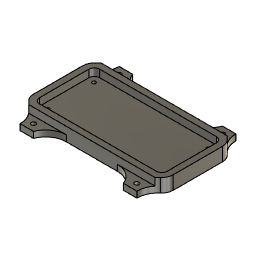
amod3-electronics_platform v9 (Autodesk Fusion 360 archive; units mm, degrees)
design "amod3-px_holder"
Autodesk Fusion 360 part; units mm, degrees
sketch "Sketch1" plane through (0, 0, 0) normal (0, 0, 1) x (1, 0, 0)
  line L0 (-21, 0) -> (65.86, 0)
  line L1 (69.86, 4) -> (69.86, 40.69)
  line L2 (65.86, 44.69) -> (-21, 44.69)
  line L3 (-25, 40.69) -> (-25, 4)
  arc A0 (-21, 44.69) -> (-25, 40.69) centre (-21, 40.69) ccw
  arc A1 (-25, 4) -> (-21, 0) centre (-21, 4) ccw
  arc A2 (69.86, 40.69) -> (65.86, 44.69) centre (65.86, 40.69) ccw
  arc A3 (65.86, 0) -> (69.86, 4) centre (65.86, 4) ccw
  line L4 (-25, 44.69) -> (69.86, 0)
  line L5 (69.86, 0) -> (69.86, 44.69)
  line L6 (69.86, 44.69) -> (-25, 0)
  line L7 (64.93, 5.145) -> (-20.07, 5.145)
  line L8 (-20.07, 5.145) -> (-20.07, 39.545)
  line L9 (-20.07, 39.545) -> (64.93, 39.545)
  line L10 (64.93, 39.545) -> (64.93, 5.145)
  line L11 (64.93, 5.145) -> (-20.07, 39.545) construction
  line L12 (-20.07, 5.145) -> (64.93, 39.545) construction
  circle A4 centre (-20.07, 39.545) radius 1.35
  circle A5 centre (64.93, 39.545) radius 1.35
  circle A6 centre (-20.07, 5.145) radius 1.35
  circle A7 centre (64.93, 5.145) radius 1.35
  line L13 (-29.5, 40.69) -> (-29.5, 4)
  arc A8 (-29.5, 4) -> (-21, -4.5) centre (-21, 4) ccw
  line L14 (-21, -4.5) -> (65.86, -4.5)
  arc A9 (65.86, -4.5) -> (74.36, 4) centre (65.86, 4) ccw
  line L15 (74.36, 4) -> (74.36, 40.69)
  arc A10 (74.36, 40.69) -> (65.86, 49.19) centre (65.86, 40.69) ccw
  line L16 (65.86, 49.19) -> (-21, 49.19)
  arc A11 (-21, 49.19) -> (-29.5, 40.69) centre (-21, 40.69) ccw
  circle A12 centre (-20.07, 5.145) radius 2.6
  circle A13 centre (64.93, 5.145) radius 2.6
  circle A14 centre (-20.07, 39.545) radius 2.6
  circle A15 centre (64.93, 39.545) radius 2.6
  line L17 (-21, -4.5) -> (-11, -4.5)
  line L18 (-11, -4.5) -> (-11, -14.5)
  line L19 (-11, -14.5) -> (-21, -14.5)
  line L20 (-21, -14.5) -> (-21, -4.5)
  line L21 (-11, -4.5) -> (-21, -4.5)
  line L22 (65.86, -4.5) -> (55.86, -4.5)
  line L23 (65.86, -4.5) -> (65.86, -14.5)
  line L24 (65.86, -14.5) -> (55.86, -14.5)
  line L25 (55.86, -14.5) -> (55.86, -4.5)
  line L26 (-11, 59.19) -> (-21, 59.19)
  line L27 (-11, 59.19) -> (-11, 49.19)
  line L28 (-11, 49.19) -> (-21, 49.19)
  line L29 (-21, 49.19) -> (-21, 59.19)
  line L30 (65.86, 59.19) -> (55.86, 59.19)
  line L31 (65.86, 59.19) -> (65.86, 49.19)
  line L32 (65.86, 49.19) -> (55.86, 49.19)
  line L33 (55.86, 49.19) -> (55.86, 59.19)
  point P0 (-25, 0)
  point P1 (69.86, 0)
  point P2 (-25, 44.69)
  point P3 (22.43, 22.345)
  dimension "d1" = 94.86
  dimension "d2" = 44.69
  dimension "d3" = 4
  dimension "d4" = 4
  dimension "d5" = 4
  dimension "d6" = 4
  dimension "d7" = 85
  dimension "d8" = 34.4
  dimension "d9" = 2.7
  dimension "d12" = 85
  dimension "d13" = -34.4
  dimension "d14" = 4.5
  dimension "d19" = 5.2
  dimension "d22" = 85
  dimension "d23" = 34.4
  dimension "d28" = 10
  dimension "d29" = 10
  dimension "d32" = 76.86
  dimension "d33" = 63.69
  constraint horizontal L0
  constraint vertical L1
  constraint horizontal L2
  constraint vertical L3
  constraint coincident P2 L2
  constraint coincident P2 L3
  constraint tangent L2 A0
  constraint tangent L3 A0
  constraint coincident P0 L0
  constraint coincident P0 L3
  constraint tangent L0 A1
  constraint tangent L3 A1
  constraint tangent L1 A2
  constraint tangent L2 A2
  constraint coincident P1 L0
  constraint coincident P1 L1
  constraint tangent L0 A3
  constraint tangent L1 A3
  constraint coincident P2 L4.start
  constraint coincident P1 L4.end
  constraint vertical L5
  constraint coincident P0 L6.end
  constraint horizontal L7
  constraint perpendicular L7 L8
  constraint parallel L7 L9
  constraint parallel L8 L10
  constraint coincident L11 P3
  constraint coincident L12 P3
  constraint midpoint L4 P3
  constraint coincident L8.end L9.start
  constraint concentric A6 A12
  constraint horizontal L17
  constraint vertical L18
  constraint horizontal L19
  constraint vertical L20
  measures "d1" distance of P0 L4.end
  measures "d2" distance of P0 P2
  measures "d3" radius of A0
  measures "d4" radius of A1
  measures "d5" radius of A2
  measures "d6" radius of A3
  measures "d7" distance of L8.end L9.end
  measures "d8" distance of L7.end L8.end
  measures "d9" diameter of A4
  measures "d19" diameter of A12
  measures "d28" distance of A8.end L17.end
  measures "d29" distance of A8.end L19.end
extrude "Extrude1" add sketch "Sketch1" along normal blind 10 contours A3 L4 L5 | A2 L5 L6 | L13 A8 L14 A9 L15 A10 L16 A11 L17 L21 L22 L28 L32
extrude "Extrude2" add sketch "Sketch1" along normal blind 3 contours L0 A1 A3 L4 L6 L7 A12 A13 | L3 A0 A1 L4 L6 L8 A12 A14 | L1 A2 A3 L4 L5 L6 L10 A13 A15 | L6 L7 L8 A6 A12 | L6 A12 | L4 A13 | L4 L7 L10 A7 A13 | L6 L7 A12 | L7 L8 A6 A12 | L4 L6 L7 L8 L9 A12 A14 | L4 L7 A13 | L2 A0 A2 L4 L6 L9 A14 A15 | L4 L6 L7 | L4 L8 L9 A4 A14 | L8 L9 A4 A14 | L4 L6 L7 L9 L10 A13 A15 | L7 L10 A7 A13 | L4 A14 | L4 L6 L9 | L4 L9 A14 | L6 L9 L10 A5 A15 | L6 A15 | L9 L10 A5 A15 | L6 L9 A15
sketch "Sketch2" plane through (0, 0, 0) normal (0, 0, 1) x (1, 0, 0)
extrude "Extrude3" cut sketch "Sketch1" along normal blind 2.5 contours L6 L7 L8 A6 A12 | L4 L7 L10 A7 A13 | L7 L8 A6 A12 | L4 L8 L9 A4 A14 | L8 L9 A4 A14 | L7 L10 A7 A13 | L6 L9 L10 A5 A15 | L9 L10 A5 A15
extrude "Extrude4" add 1 faces at (36.1652, 16.8113, 3) along direction (0, 0, 1) blind 1.5
extrude "Extrude5" add sketch "Sketch1" along normal blind 4.5 contours L16 L26 L27 L28 L29 | L14 L17 L18 L19 L20 L21 | L16 L30 L31 L32 L33 | L14 L22 L23 L24 L25
sketch "Sketch3" plane through (0, 0, 0) normal (0, 0, -1) x (1, 0, 0)
  line L0 (-18.5378, -41.6456) -> (-19.4259, -42.064)
  arc A0 (-18.5378, -41.6456) -> (-19.4259, -42.064) centre (-20.07, -39.545) ccw
  line L1 (64.2859, -42.064) -> (63.3978, -41.6456)
  arc A1 (64.2859, -42.064) -> (63.3978, -41.6456) centre (64.93, -39.545) ccw
  line L2 (-19.4259, -2.626) -> (-18.5378, -3.0444)
  arc A2 (-19.4259, -2.626) -> (-18.5378, -3.0444) centre (-20.07, -5.145) ccw
  line L3 (63.3978, -3.0444) -> (64.2859, -2.626)
  arc A3 (63.3978, -3.0444) -> (64.2859, -2.626) centre (64.93, -5.145) ccw
  arc A4 (-29.5, -40.69) -> (-21, -49.19) centre (-21, -40.69) ccw
  line L4 (-21, -49.19) -> (-21, -59.19)
  line L5 (-21, -59.19) -> (-11, -59.19)
  line L6 (-11, -59.19) -> (-11, -49.19)
  line L7 (-11, -49.19) -> (55.86, -49.19)
  line L8 (55.86, -49.19) -> (55.86, -59.19)
  line L9 (55.86, -59.19) -> (65.86, -59.19)
  line L10 (65.86, -59.19) -> (65.86, -49.19)
  arc A5 (65.86, -49.19) -> (74.36, -40.69) centre (65.86, -40.69) ccw
  line L11 (74.36, -40.69) -> (74.36, -4)
  arc A6 (74.36, -4) -> (65.86, 4.5) centre (65.86, -4) ccw
  line L12 (65.86, 4.5) -> (65.86, 14.5)
  line L13 (65.86, 14.5) -> (55.86, 14.5)
  line L14 (55.86, 14.5) -> (55.86, 4.5)
  line L15 (55.86, 4.5) -> (-11, 4.5)
  line L16 (-11, 4.5) -> (-11, 14.5)
  line L17 (-11, 14.5) -> (-21, 14.5)
  line L18 (-21, 14.5) -> (-21, 4.5)
  arc A7 (-21, 4.5) -> (-29.5, -4) centre (-21, -4) ccw
  line L19 (-29.5, -4) -> (-29.5, -40.69)
  line L20 (-21, 14.5) -> (65.86, 14.5)
  line L21 (65.86, 14.5) -> (65.86, -59.19)
  line L22 (65.86, -59.19) -> (-21, -59.19)
  line L23 (-21, -59.19) -> (-21, 14.5)
  line L24 (-11, 4.5) -> (55.86, 4.5)
  line L25 (55.86, 4.5) -> (55.86, -49.19)
  line L26 (55.86, -49.19) -> (-11, -49.19)
  line L27 (-11, -49.19) -> (-11, 4.5)
  line L28 (-11, 4.5) -> (-21, 14.5)
  line L29 (55.86, 4.5) -> (65.86, 14.5)
  line L30 (55.86, -49.19) -> (65.86, -59.19)
  line L31 (-11, -49.19) -> (-21, -59.19)
  circle A8 centre (-16, 9.5) radius 1.65
  circle A9 centre (60.86, 9.5) radius 1.65
  circle A10 centre (-16, -54.19) radius 1.65
  circle A11 centre (60.86, -54.19) radius 1.65
  dimension "d36" = 3.3
  dimension "d37" = 3.3
  dimension "d38" = 3.3
  dimension "d39" = 3.3
  constraint horizontal L20
  constraint vertical L21
  constraint horizontal L22
  constraint vertical L23
  constraint coincident L9.end L10.start
  constraint coincident L17.end L18.start
  constraint horizontal L24
  constraint vertical L25
  constraint horizontal L26
  constraint vertical L27
  constraint coincident L7.end L8.start
  constraint coincident L15.end L16.start
  constraint coincident L14.end L15.start
  constraint coincident L12.end L13.start
  constraint coincident L6.end L7.start
  constraint coincident L4.end L5.start
  constraint midpoint L28 A8.centre
  constraint midpoint L29 A9.centre
  constraint midpoint L31 A10.centre
  constraint midpoint L30 A11.centre
  measures "d36" diameter of A8
  measures "d37" diameter of A9
  measures "d38" diameter of A10
  measures "d39" diameter of A11
extrude "Extrude6" cut sketch "Sketch3" against normal blind 8.5 contours L31 A10 | L31 A10 | L28 A8 | L28 A8 | L30 A11 | L30 A11 | L29 A9 | L29 A9
fillet "Fillet1" radius 15.5 8 edges at (-21, -4.5, 2.25) (55.86, -4.5, 2.25) (-11, -4.5, 2.25) (65.86, -4.5, 2.25) (-11, 49.19, 2.25) (65.86, 49.19, 2.25) (55.86, 49.19, 2.25) (-21, 49.19, 2.25)
